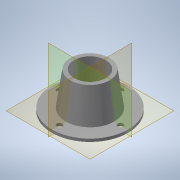
# Autodesk Inventor part: DC motor connectie
Saved by Autodesk Inventor 2021 (Build 250183000, 183)
## iProperties
Manager: PJ / DCS
Company: Emmaüs Bovenbouw Aalter
Created: 2021-01-09
Part Number: DC motor connectie
Material: S235
Catalog Web Link: http://emmausbovenbouw.op-weg.be/
Vendor: Emmaüsinstituut Bovenbouw Aalter
Document SubType Name: Modeling
Designer: Antho
Engineer: Declercq St.
Manufacturer: Standard
Standards Organization: Custom
Density: 7.86 g/cm^3
Appearance: Steel
Title: Algemene titel
Subject: Specifieke titel
Author: Antho
Keywords: Ruwe Ø xxxxx
Comments: Opmerking
Autodesk Inventor part; units mm, degrees
sketch "Sketch1" plane through (0, 0, 0) normal (0, 0, 1) x (1, 0, 0)
  line L0 (0, 2.8582) -> (0, -2.8582) construction
  line L1 (-5.7775, 0) -> (5.7775, 0) construction
  circle A0 centre (0, 0) radius 5.75
  circle A1 centre (0, 0) radius 3.5
  circle A2 centre (0, 0) radius 20
  dimension "d0" = 11.5
  dimension "d1" = 7
  dimension "d2" = 40
  constraints: 4 coincident, 4 end point, 3 centre point, 2 midpoint, 1 horizontal, 1 vertical
  measures "d0" diameter of A0
  measures "d1" diameter of A1
  measures "d2" diameter of A2
extrude "Extrusion1" add sketch "Sketch1" along normal blind 1.5 contours A0 | A2
sketch "Sketch2" plane through (0, 0, 1.5) normal (0, 0, 1) x (1, 0, 0)
  circle A0 centre (0, 0) radius 8.25
  circle A1 centre (0, 0) radius 10.25
  dimension "d5" = 16.5
  dimension "d6" = 20.5
  constraints: 2 centre point, 2 coincident
  measures "d5" diameter of A0
  measures "d6" diameter of A1
extrude "Extrusion2" add sketch "Sketch2" along normal blind 17.5
sketch "Sketch4" plane through (0, 0, 1.5) normal (0, 0, 1) x (1, 0, 0)
  circle A0 centre (0, 0) radius 20 projected
  line L0 (0, 0) -> (0, 16)
  line L1 (0, 0) -> (16, 0)
  line L2 (0, 0) -> (0, -16)
  line L3 (0, 0) -> (-16, 0)
  dimension "d9" = 16
  dimension "d10" = 16
  dimension "d11" = 16
  dimension "d12" = 16
  constraints: 8 end point, 4 coincident, 2 horizontal, 2 vertical
  measures "d9" distance of L0.start L0.end
  measures "d10" distance of L0.start L1.end
  measures "d11" distance of L0.start L2.end
  measures "d12" distance of L0.start L3.end
hole "Hole1" at (0, 16, 1.5) at (16, 0, 1.5) at (0, -16, 1.5) at (-16, 0, 1.5) direction (0, 0, -1) diameter 3 depth 1.5
draft "FaceDraft2" angle 8 pull direction (0, 0, 1) faces at (10.2168, -0.8248, 13.1667) fixed edges at (-10.25, 0, 19)
body "Solid1"
